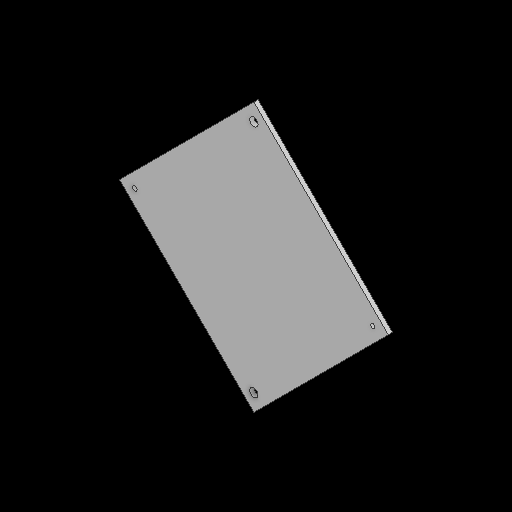
# Autodesk Inventor part: z_plate
Saved by Autodesk Inventor 2026.1 (Build 301233000, 233)
## iProperties
Created: 2025-09-21
Part Number: z_plate
Material: Generic
Document SubType Name: Modeling
Designer: drago
Density: 1 g/cm^3
Appearance: Default
Author: drago
Autodesk Inventor part; units mm, degrees
ref_plane "YZ Plane" through (0, 0, 0) normal (1, 0, 0) x (0, 1, 0)
ref_plane "XZ Plane" through (0, 0, 0) normal (0, 1, 0) x (-1, 0, 0)
ref_plane "XY Plane" through (0, 0, 0) normal (0, 0, 1) x (1, 0, 0)
sketch "Sketch1" plane through (0, 0, 0) normal (0, 0, 1) x (1, 0, 0)
  circle A0 centre (281.7, 0) radius 5.25
  circle A1 centre (-281.7, 0) radius 5.25
  circle A2 centre (0, 277.5) radius 10
  circle A3 centre (0, -277.5) radius 10
  line L0 (0, -318.1981) -> (318.1981, 0)
  line L1 (318.1981, 0) -> (0, 318.1981)
  line L2 (0, 318.1981) -> (-318.1981, 0)
  line L3 (-318.1981, 0) -> (0, -318.1981)
  line L4 (0, -318.1981) -> (0, 318.1981) construction
  line L5 (318.1981, 0) -> (-318.1981, 0) construction
  line L6 (0, -318.1981) -> (450, -318.1981) construction
  point P0 (0, 0)
  point P1 (0, 0)
  point P2 (0, 0)
  dimension "d5" = 10.5
  dimension "d6" = 281.7
  dimension "d7" = 10.5
  dimension "d9" = 281.7
  dimension "d10" = 20
  dimension "d11" = 20
  dimension "d12" = 277.5
  dimension "d13" = 277.5
  dimension "d14" = 450
  dimension "d15" = 45
  dimension "d16" = 450
  constraints: 14 end point, 4 centre point, 2 midpoint, 2 parallel, 1 equal length, 1 horizontal, 1 perpendicular
  measures "d5" diameter of A0
  measures "d6" distance of point (0, 0) A0.centre
  measures "d7" diameter of A1
  measures "d9" distance of point (0, 0) A1.centre
  measures "d10" diameter of A2
  measures "d11" diameter of A3
  measures "d12" distance of A3.centre point (0, 0)
  measures "d13" distance of point (0, 0) A2.centre
  measures "d14" distance of L0.start L0.end
  measures "d15" angle of L6 L0
  measures "d16" distance of L1.end L0.end
extrude "Extrusion1" add sketch "Sketch1" against normal blind 10
equation "\"d5\" = diam_leadscrew_hole"
equation "\"d6\" = 0.5 * diag_dist_leadscrews"
equation "\"d7\" = diam_leadscrew_hole"
equation "\"d9\" = 0.5 * diag_dist_leadscrews"
equation "\"d10\" = diam_rail_hole"
equation "\"d11\" = diam_rail_hole"
equation "\"d12\" = 0.5 * diag_dist_rails"
equation "\"d13\" = 0.5 * diag_dist_rails"
equation "\"d14\" = z_plate_width"
equation "\"d16\" = z_plate_width"
equation "\"diag_dist_rails\" = 555"
equation "\"diag_dist_leadscrews\" = 563.4"
equation "\"diam_leadscrew_hole\" = 10.5"
equation "\"diam_rail_hole\" = 20"
equation "\"z_plate_width\" = 450"
body "Solid1"
